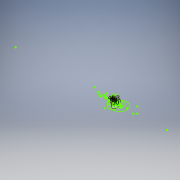
# Autodesk Inventor part: cSkull_meso_WOK_tall_VIS
Saved by Autodesk Inventor 2018 (Build 220112000, 112)
## iProperties
Created: 2018-05-22
Part Number: cSkull_meso_WOK_tall_VIS
Material: Generic
Document SubType Name: Modeling
Designer: McCormick Lab
Density: 1 g/cm^3
Appearance: Default
Author: McCormick Lab
Autodesk Inventor part; units mm, degrees
ref_plane "YZ Plane" through (0, 0, 0) normal (1, 0, 0) x (0, 1, 0)
ref_plane "XZ Plane" through (0, 0, 0) normal (0, 1, 0) x (-1, 0, 0)
ref_plane "XY Plane" through (0, 0, 0) normal (0, 0, 1) x (1, 0, 0)
sketch "Sketch1" plane through (0, 0, 0) normal (1, 0, 0) x (0, 1, 0)
  arc A0 (6, 5) -> (0, 6.4776) centre (1.5083, -0.3184) ccw
  arc A1 (0, 6.4776) -> (-6, 2) centre (-0.0372, 0.2686) ccw
  arc A2 (-6, 2) -> (-5, -3.4628) centre (-1.5043, 0) ccw
  arc A3 (-5, -3.4628) -> (2, -5.5969) centre (1.6627, 5.8444) ccw
  arc A4 (2, -5.5969) -> (6.9353, -3.4628) centre (1.5482, 2.2219) ccw
  arc A5 (6, 5) -> (13, 1) centre (22.0402, 24.9454) ccw
  arc A6 (13, -1) -> (6.9353, -3.4628) centre (16.5953, -18.5517) ccw
  arc A7 (13, -1) -> (13, 1) centre (11.912, 0) ccw
  arc A8 (15.1251, -1.2068) -> (15.1251, 1.1192) centre (13.8597, -0.0438) ccw
  arc A9 (6.9841, 5.7712) -> (15.1251, 1.1192) centre (25.6388, 28.9677) ccw
  arc A10 (6.9841, 5.7712) -> (0.0061, 7.4897) centre (1.7602, -0.414) ccw
  arc A11 (0.0061, 7.4897) -> (-6.9719, 2.2822) centre (-0.0372, 0.2686) ccw
  arc A12 (-6.9719, 2.2822) -> (-5.8089, -4.0711) centre (-1.7435, -0.0438) ccw
  arc A13 (-5.8089, -4.0711) -> (2.3321, -6.5529) centre (1.9397, 6.7532) ccw
  arc A14 (2.3321, -6.5529) -> (8.0718, -4.0711) centre (1.8067, 2.5403) ccw
  arc A15 (15.1251, -1.2068) -> (8.0718, -4.0711) centre (19.3063, -21.6193) ccw
  point P0 (0, 0)
  constraints: 32 point on circle, 16 centre point
sketch "Sketch2" plane through (0, 0, 0) normal (0, 0, 1) x (1, 0, 0)
  arc A0 (4.5893, 15.6275) -> (5.3653, 12.7341) centre (8.4769, 15.1194) ccw
  arc A1 (7.1334, 6.0475) -> (5.3653, 12.7341) centre (-9.3019, 5.2787) ccw
  arc A2 (4, -1) -> (7.1334, 6.0475) centre (-2.3212, 6.0308) ccw
  arc A3 (4, -1) -> (2.2783, -7.605) centre (15.174, -7.4395) ccw
  arc A4 (4.5893, 15.6275) -> (-5.4042, 15.6275) centre (-0.4074, 13.9881) ccw
  arc A5 (-4.7137, -7.4395) -> (2.2783, -7.605) centre (-1.0169, 0.9638) ccw
  arc A6 (-5.4042, 15.6275) -> (-4.7137, -7.4395) centre (15.8945, 4.7212) ccw
  point P0 (0, 0)
  point P1 (16.0644, 6.0537)
  constraints: 14 point on circle, 7 centre point
sketch "Sketch3" plane through (0, 0, 0) normal (0, 0, 1) x (1, 0, 0)
  line L0 (8, 6) -> (8, -9.7213)
  line L1 (8, 6) -> (8, 19.0901)
  arc A0 (8, -9.7213) -> (8, 19.0901) centre (-3.1204, 4.6844) ccw
  point P0 (0, 0)
  constraints: 4 end point, 2 point on circle, 1 centre point, 1 vertical
sketch "Sketch4" plane through (0, 0, 0) normal (0, 0, 1) x (1, 0, 0)
  arc A0 (4, -3) -> (3, -7.466) centre (10.199, -6.733) ccw
  arc A1 (4, -3) -> (7.6292, 3.7812) centre (-12.6955, 10.297) ccw
  arc A2 (7.6292, 3.7812) -> (7, 11) centre (-7.2238, 6.1234) ccw
  arc A3 (7, 11) -> (6.1482, 13) centre (-7.2238, 6.1234) ccw
  arc A4 (5.3976, 15.5783) -> (6.1482, 13) centre (8.6756, 15.1342) ccw
  arc A5 (3, -7.466) -> (9, -9) centre (8, -0.4104) ccw
  arc A6 (11, 18) -> (5.3976, 15.5783) centre (10.5, 11.4654) ccw
  arc A7 (9, -9) -> (11, 18) centre (-69.2967, 10.3738) ccw
  point P0 (0, 0)
  constraints: 16 point on circle, 8 centre point
sketch "Sketch5" plane through (0, 0, 0) normal (1, 0, 0) x (0, 1, 0)
  arc A0 (13, -1.7602) -> (13, 2.0171) centre (12.6189, 0.1284) ccw
  arc A1 (17, 0) -> (13, 2.0171) centre (12.9569, -3.0431) ccw
  arc A2 (13, -1.7602) -> (17, 0) centre (13.7728, 1.9087) ccw
  point P0 (0, 0)
  constraints: 6 point on circle, 3 centre point
sketch "Sketch7" plane through (0, 0, 0) normal (1, 0, 0) x (0, 1, 0)
  circle A0 centre (5, 0.3375) radius 25
  point P0 (0, 0)
  dimension "d10" = 50
  constraints: 1 centre point
  measures "d10" diameter of A0
sketch "Sketch8" plane through (0, 0, 0) normal (0, 0, 1) x (1, 0, 0)
  arc A0 (4.5893, 15.6275) -> (5.3653, 12.7341) centre (8.4769, 15.1194) ccw
  arc A1 (7.1334, 6.0475) -> (5.3653, 12.7341) centre (-9.3019, 5.2787) ccw
  arc A2 (4, -1) -> (7.1334, 6.0475) centre (-2.3212, 6.0308) ccw
  arc A3 (4, -1) -> (2.2783, -7.605) centre (15.174, -7.4395) ccw
  arc A4 (4.5893, 15.6275) -> (-5.4042, 15.6275) centre (-0.4074, 13.9881) ccw
  arc A5 (-4.7137, -7.4395) -> (2.2783, -7.605) centre (-1.0169, 0.9638) ccw
  arc A6 (-5.4042, 15.6275) -> (-4.7137, -7.4395) centre (15.8945, 4.7212) ccw
  point P0 (0, 0)
  constraints: 14 point on circle, 7 centre point
sketch "Sketch9" plane through (0, 0, 0) normal (0, 0, 1) x (1, 0, 0)
  line L0 (2.2936, -15.8564) -> (2.2936, -6.8564)
  arc A0 (2.2936, -6.8564) -> (-3.9962, -9.9765) centre (0.2723, -10.6815) ccw
  arc A1 (-4, -16) -> (2.2936, -15.8564) centre (-0.9465, -11.8394) ccw
  arc A2 (-3.9962, -9.9765) -> (-4, -16) centre (14.3076, -12.9998) ccw
  point P0 (0, 0)
  constraints: 6 point on circle, 3 centre point, 2 end point, 1 tangent
sketch "Sketch10" plane through (0, 0, 0) normal (1, 0, 0) x (0, 1, 0)
  arc A0 (13, -1) -> (13, 1) centre (11.912, 0) ccw
  arc A1 (6, 5) -> (13, 1) centre (22.0402, 24.9454) ccw
  arc A2 (6, 5) -> (0, 6.4776) centre (1.5083, -0.3184) ccw
  arc A3 (0, 6.4776) -> (-6, 2) centre (-0.0372, 0.2686) ccw
  arc A4 (-6, 2) -> (-5, -3.4628) centre (-1.5043, 0) ccw
  arc A5 (-5, -3.4628) -> (2, -5.5969) centre (1.6627, 5.8444) ccw
  arc A6 (2, -5.5969) -> (6.9353, -3.4628) centre (1.5482, 2.2219) ccw
  arc A7 (13, -1) -> (6.9353, -3.4628) centre (16.5953, -18.5517) ccw
  point P0 (0, 0)
  constraints: 16 point on circle, 8 centre point
sketch "Sketch11" plane through (0, 0, 0) normal (0, 0, 1) x (1, 0, 0)
  arc A0 (4, -3) -> (3, -7.466) centre (10.199, -6.733) ccw
  arc A1 (4, -3) -> (7.6292, 3.7812) centre (-12.6955, 10.297) ccw
  arc A2 (7.6292, 3.7812) -> (7, 11) centre (-7.2238, 6.1234) ccw
  arc A3 (7, 11) -> (6.1482, 13) centre (-7.2238, 6.1234) ccw
  arc A4 (5.3976, 15.5783) -> (6.1482, 13) centre (8.6756, 15.1342) ccw
  arc A5 (11, -15) -> (11, 18) centre (-58.5, 1.5) ccw
  arc A6 (3, -7.466) -> (3.1376, -15) centre (85.1776, -9.733) ccw
  arc A7 (6, 24) -> (5.3976, 15.5783) centre (36.0186, 17.6203) ccw
  arc A8 (11, 18) -> (6, 24) centre (2.7033, 16.1694) ccw
  arc A9 (3.1376, -15) -> (11, -15) centre (7.0688, -10.5838) ccw
  arc A10 (5, 24) -> (4.5969, 15.5783) centre (45.756, 17.829) ccw
  arc A11 (-2, 19) -> (4.5969, 15.5783) centre (5.6189, 25.6189) ccw
  arc A12 (5, 24) -> (-2, 19) centre (11.5, 7.5) ccw
  point P0 (0, 0)
  constraints: 26 point on circle, 13 centre point
sketch "Sketch12" plane through (0, 0, 0) normal (1, 0, 0) x (0, 1, 0)
  circle A0 centre (3, 0.2318) radius 20
  circle A1 centre (3, 0.2318) radius 19
  point P0 (0, 0)
  dimension "d21" = 40
  dimension "d22" = 38
  constraints: 2 centre point, 1 coincident
  measures "d21" diameter of A0
  measures "d22" diameter of A1
sketch "Sketch13" plane through (0, 0, 0) normal (0, 0, 1) x (1, 0, 0)
  arc A0 (4.6444, -3) -> (3.6444, -7.466) centre (10.8434, -6.733) ccw
  arc A1 (4.6444, -3) -> (8.2736, 3.7812) centre (-12.0511, 10.297) ccw
  arc A2 (8.2736, 3.7812) -> (7.6444, 11) centre (-6.5793, 6.1234) ccw
  arc A3 (7.6444, 11) -> (6.7926, 13) centre (-6.5793, 6.1234) ccw
  arc A4 (6.042, 15.5783) -> (6.7926, 13) centre (9.3201, 15.1342) ccw
  arc A5 (12.1446, -13.3563) -> (11.6094, 18.8213) centre (-67.1488, 1.418) ccw
  arc A6 (4.5893, 15.6275) -> (5.3653, 12.7341) centre (8.4769, 15.1194) ccw
  arc A7 (7.1334, 6.0475) -> (5.3653, 12.7341) centre (-9.3019, 5.2787) ccw
  arc A8 (4, -1) -> (7.1334, 6.0475) centre (-2.3212, 6.0308) ccw
  arc A9 (4, -1) -> (2.2783, -7.605) centre (15.174, -7.4395) ccw
  arc A10 (-5.4042, 15.6275) -> (-4.7137, -7.4395) centre (15.8945, 4.7212) ccw
  arc A11 (3.6444, -7.466) -> (4.6444, -19) centre (48.1921, -9.4141) ccw
  arc A12 (1, -17) -> (2.2783, -7.605) centre (-20.1318, -9.3402) ccw
  arc A13 (4.5893, 15.6275) -> (4, 28) centre (-90.183, 17.3138) ccw
  arc A14 (6.0097, 28) -> (6.042, 15.5783) centre (472.3708, 23) ccw
  arc A15 (4.6444, -19) -> (12.1446, -13.3563) centre (5.8088, -12.7419) ccw
  arc A16 (11.6094, 18.8213) -> (6.0097, 28) centre (-7.4499, 13.4913) ccw
  arc A17 (-4.7137, -7.4395) -> (1, -17) centre (32.2099, 8.14) ccw
  arc A18 (4, 28) -> (-5.4042, 15.6275) centre (39.2165, -8.5279) ccw
  point P0 (0, 0)
  constraints: 38 point on circle, 19 centre point
sketch "Sketch16" plane through (0, 0, 0) normal (0, 0, 1) x (1, 0, 0)
  arc A0 (7.7852, 10.9763) -> (6.9451, 12.9812) centre (-6.467, 6.1832) ccw
  arc A1 (8.372, 3.7539) -> (7.7852, 10.9763) centre (-6.467, 6.1832) ccw
  arc A2 (4.7031, -3.0059) -> (8.372, 3.7539) centre (-11.9141, 10.3888) ccw
  arc A3 (4.7031, -3.0059) -> (3.6769, -7.4659) centre (10.88, -6.7752) ccw
  arc A4 (6.2096, 15.5639) -> (6.9451, 12.9812) centre (9.485, 15.1006) ccw
  line L0 (3.6769, -7.4659) -> (3.6769, -13)
  line L1 (3.6769, -13) -> (8.7312, -13)
  line L2 (7.1813, -23) -> (8.45, -23) projected
  line L3 (6.2096, 15.5639) -> (6.0634, 19)
  line L4 (6.0634, 19) -> (8.7312, 19)
  line L5 (8.7312, 19) -> (8.7312, -13)
  point P0 (0, 0)
  constraints: 10 end point, 10 point on circle, 5 centre point, 1 parallel, 1 vertical
sketch "Sketch18" plane through (0, 0, 0) normal (0, 1, 0) x (-1, 0, 0)
  arc A0 (0, 16) -> (0, -16) centre (63, 0) ccw
  arc A1 (0, -16) -> (0, 16) centre (-1, 0) ccw
  point P0 (0, 0)
  constraints: 4 point on circle, 2 centre point
sketch "Sketch19" plane through (0, 0, 0) normal (0, 0, 1) x (1, 0, 0)
  arc A0 (0, -13) -> (0, 21.2939) centre (-44.6367, 4.1469) ccw
  arc A1 (0, 21.2939) -> (0, -13) centre (9.2646, 4.1469) ccw
  point P0 (0, 0)
  constraints: 4 point on circle, 2 centre point
sketch "Sketch20" plane through (0, 0, 0) normal (0, 1, 0) x (-1, 0, 0)
  arc A0 (0, 18) -> (0, -21) centre (116.9496, -1.5) ccw
  arc A1 (0, -21) -> (0, 18) centre (-188.5, -1.5) ccw
  point P0 (0, 0)
  constraints: 4 point on circle, 2 centre point
sketch "Sketch21" plane through (0, 0, 0) normal (0, 0, 1) x (1, 0, 0)
  arc A0 (4.5893, 15.6275) -> (5.3653, 12.7341) centre (8.4769, 15.1194) ccw
  arc A1 (7.1334, 6.0475) -> (5.3653, 12.7341) centre (-9.3019, 5.2787) ccw
  arc A2 (4, -1) -> (7.1334, 6.0475) centre (-2.3212, 6.0308) ccw
  arc A3 (4, -1) -> (2.2783, -7.605) centre (15.174, -7.4395) ccw
  arc A4 (-5.4042, 15.6275) -> (-4.7137, -7.4395) centre (15.8945, 4.7212) ccw
  arc A5 (1.6146, -47) -> (2.2783, -7.605) centre (-871.3055, -12.5889) ccw
  arc A6 (-4.7137, -7.4395) -> (1.6146, -47) centre (3.6662, -26.3854) ccw
  arc A7 (6.6047, 48.2766) -> (4.5893, 15.6275) centre (207.8183, 19.4692) ccw
  arc A8 (6.6047, 48.2766) -> (-5.4042, 15.6275) centre (18.1068, 25.5128) ccw
  point P0 (4.9602, 0)
  constraints: 18 point on circle, 9 centre point
sketch "Sketch22" plane through (0, 0, 0) normal (1, 0, 0) x (0, 1, 0)
  arc A0 (12.671, -1.508) -> (10.1452, -2.4415) centre (13.2273, -6.897) ccw
  arc A1 (5.972, -5.9193) -> (10.1452, -2.4415) centre (1.4729, 3.7221) ccw
  arc A2 (-1.0034, -7.134) -> (5.972, -5.9193) centre (0.0411, 7.5036) ccw
  arc A3 (-6.1623, -3.0965) -> (-1.0034, -7.134) centre (-0.5861, -1.2862) ccw
  arc A4 (-5.468, 3.7221) -> (-6.1623, -3.0965) centre (0.6002, -0.3405) ccw
  arc A5 (6.5632, 5.6579) -> (-0.5861, 6.5886) centre (1.6095, -4.4698) ccw
  arc A6 (-0.5861, 6.5886) -> (-5.468, 3.7221) centre (0, 0) ccw
  arc A7 (6.5632, 5.6579) -> (11.3492, 2.8919) centre (22.0985, 27.015) ccw
  arc A8 (14.2401, 1.3463) -> (11.3492, 2.8919) centre (11.1023, -1.0462) ccw
  arc A9 (13.4173, -1.2862) -> (14.2401, 1.3463) centre (12.4465, 0.462) ccw
  arc A10 (12.671, -1.508) -> (13.4173, -1.2862) centre (12.7302, -0.341) ccw
  point P0 (0, 0)
  point P1 (20.1069, -9.3097)
  constraints: 22 point on circle, 11 centre point, 1 tangent
sketch "Sketch23" plane through (0, 0, 0) normal (0, 0, 1) x (1, 0, 0)
  arc A0 (4, -3) -> (3, -7.466) centre (10.199, -6.733) ccw
  arc A1 (4, -3) -> (7.6292, 3.7812) centre (-12.6955, 10.297) ccw
  arc A2 (7.6292, 3.7812) -> (7, 11) centre (-7.2238, 6.1234) ccw
  arc A3 (7, 11) -> (6.1482, 13) centre (-7.2238, 6.1234) ccw
  arc A4 (5.3976, 15.5783) -> (6.1482, 13) centre (8.6756, 15.1342) ccw
  arc A5 (3, -7.466) -> (12.0039, -34.009) centre (74.5087, 1.9925) ccw
  arc A6 (12.0039, -34.009) -> (12.0039, 40.009) centre (-50.8687, 3) ccw
  arc A7 (12.0039, 40.009) -> (5.3976, 15.5783) centre (75.5489, 9.7171) ccw
  point P0 (0, 0)
  constraints: 16 point on circle, 8 centre point
sketch "Sketch24" plane through (0, 0, 0) normal (1, 0, 0) x (0, 1, 0)
  circle A0 centre (4, 0) radius 24.0208
  circle A1 centre (4, 0) radius 54.037
  point P0 (0, 0)
  constraints: 2 centre point, 1 coincident
sketch "Sketch25" plane through (0, 0, 0) normal (0, 0, 1) x (1, 0, 0)
  line L0 (2.9628, -6.7024) -> (3, -28)
  arc A0 (7, 36) -> (4.5756, 19.3965) centre (118.9772, 11.1705) ccw
  arc A1 (5.9839, 23.9235) -> (5.3976, 15.5783) centre (44.4323, 17.0293) ccw
  arc A2 (5.9839, 23.9235) -> (7, 33) centre (-89.9402, 39.2578) ccw
  arc A3 (5.3976, 15.5783) -> (7, 33) centre (-0.8843, 24.9407) ccw
  arc A4 (7, 36) -> (4.5756, 19.3965) centre (13.0884, 26.6322) ccw
  arc A5 (3, -28) -> (2.9628, -6.7024) centre (-3.3961, -17.3623) ccw
  point P0 (0, 0)
  constraints: 12 point on circle, 6 centre point, 2 end point
sketch "Sketch31" plane through (0, 0, 0) normal (1, 0, 0) x (0, 1, 0)
  circle A0 centre (4.1775, 0) radius 24.15
  circle A1 centre (4.1775, 0) radius 23
  point P0 (0, 0)
  dimension "d65" = 46
  dimension "d66" = 48.3
  constraints: 2 centre point, 1 coincident
  measures "d65" diameter of A1
  measures "d66" diameter of A0
sketch "Sketch32" plane through (0, 0, 0) normal (0, 0, 1) x (1, 0, 0)
  arc A0 (4, -1) -> (2.2783, -7.605) centre (15.174, -7.4395) ccw
  arc A1 (4, -1) -> (7.1334, 6.0475) centre (-2.3212, 6.0308) ccw
  arc A2 (7.1334, 6.0475) -> (5.3653, 12.7341) centre (-9.3019, 5.2787) ccw
  arc A3 (4.5893, 15.6275) -> (5.3653, 12.7341) centre (8.4769, 15.1194) ccw
  arc A4 (-5.4042, 15.6275) -> (-4.7137, -7.4395) centre (15.8945, 4.7212) ccw
  arc A5 (1.6146, -47) -> (2.2783, -7.605) centre (-871.3055, -12.5889) ccw
  arc A6 (-4.7137, -7.4395) -> (1.6146, -47) centre (3.6662, -26.3854) ccw
  arc A7 (6.6047, 48.2766) -> (4.5893, 15.6275) centre (207.8183, 19.4692) ccw
  arc A8 (6.6047, 48.2766) -> (-5.4042, 15.6275) centre (18.1068, 25.5128) ccw
  point P0 (0, 0)
  constraints: 18 point on circle, 9 centre point
sketch "Sketch34" plane through (0, 0, 0) normal (0, 0, 1) x (1, 0, 0)
  arc A0 (5, -4) -> (9, 6) centre (-7, 6.6) ccw
  arc A1 (5, -4) -> (4, -8) centre (10.5, -7.5) ccw
  arc A2 (4, -19.9725) -> (4, -8) centre (-95.2669, -13.9862) ccw
  arc A3 (9, 6) -> (6.6308, 15) centre (-16.4523, 4.1118) ccw
  line L0 (6.6308, 15) -> (6.6308, 28.2457)
  arc A4 (4, -19.9725) -> (6.6308, 28.2457) centre (64.4177, 0.9119) ccw
  point P0 (0, 0)
  constraints: 10 point on circle, 5 centre point, 2 end point, 1 vertical
sketch "Sketch35" plane through (0, 0, 0) normal (0, 0, 1) x (1, 0, 0)
  arc A0 (12, -8) -> (-7, -11) centre (15.0455, -88.9545) ccw
  arc A1 (-7, -11) -> (12, -8) centre (3.194, -13.8955) ccw
  point P0 (0, 0)
  constraints: 4 point on circle, 2 centre point
ref_plane "Work Plane16" through (6.6308, 4.1775, 0) normal (1, 0, 0) x (0, 0, -1)
sketch "Sketch36" plane through (6.6308, 4.1775, 0) normal (1, 0, 0) x (0, 0, -1)
  arc A0 (21.5893, 10.8225) -> (-21.5893, 10.8225) centre (0, -0.149) ccw
  arc A1 (20.2947, 10.8225) -> (-20.2947, 10.8225) centre (0, 0) ccw
  line L0 (-21.5893, 10.8225) -> (-20.2947, 10.8225)
  line L1 (-21.5893, 10.8225) -> (-20.2947, 10.8225)
  line L2 (20.2947, 10.8225) -> (21.5893, 10.8225)
  point P0 (0, -4.1775)
  constraints: 6 end point, 4 point on circle, 2 centre point, 1 horizontal
sketch "Sketch37" plane through (0, 0, 0) normal (1, 0, 0) x (0, 1, 0)
  arc A0 (15, 20.2947) -> (6, 22.9277) centre (4.1775, 0) ccw
  arc A1 (15, 21.5893) -> (6, 24.0811) centre (4.9955, 2.9543) ccw
  line L0 (15, 21.5893) -> (15, 20.2947)
  line L1 (15, 21.5893) -> (15, 20.2947)
  line L2 (6, 22.9277) -> (6, 24.0811)
  line L3 (6, 24.0811) -> (6, 22.9277)
  line L4 (15, -20.2947) -> (15, -21.5893) projected
  line L5 (15, -21.5351) -> (15, -20.2947)
  arc A2 (6, -24.0811) -> (15, -21.5893) centre (4.3914, -0.7727) ccw
  arc A3 (6, -22.9277) -> (15, -20.2947) centre (4.1775, 0) ccw
  line L6 (6, -24.0811) -> (6, -22.9277) projected
  line L7 (6, -24.0811) -> (6, -22.9277)
  point P0 (0, 0)
  constraints: 12 end point, 8 point on circle, 4 centre point, 2 collinear, 1 vertical
sketch "Sketch38" plane through (0, 0, 0) normal (0, 0, 1) x (1, 0, 0)
  arc A0 (7.1334, 6) -> (5.3972, 12.671) centre (-9.2641, 5.2939) ccw
  arc A1 (4.5581, 15) -> (5.3972, 12.671) centre (8.676, 15.1681) ccw
  line L0 (0, 15) -> (4.5581, 15) projected
  line L1 (0, 6) -> (7.1334, 6) projected
  arc A2 (4.5581, 15) -> (7.1334, 6) centre (1.4649, 9.2464) ccw
  point P0 (0, 0)
  point P1 (6.4152, 10.1452)
  point P2 (4.945, 13.4173)
  constraints: 8 point on circle, 3 centre point
sketch "Sketch39" plane through (0, 0, 0) normal (0, 0, 1) x (1, 0, 0)
  arc A0 (9, 6) -> (11.63, 15) centre (12.0023, 10.0069) ccw
  arc A1 (9, 6) -> (11.63, 15) centre (-3.4729, 14.5291) ccw
  point P0 (0, 0)
  constraints: 4 point on circle, 2 centre point
sketch "Sketch40" plane through (0, 0, 0) normal (0, 0, 1) x (1, 0, 0)
  arc A0 (1, -11) -> (5, -7) centre (4.0607, -10.0607) ccw
  arc A1 (5, -7) -> (1, -11) centre (6.5, -12.5) ccw
  point P0 (0, 0)
  point P1 (2.963, -6.7889)
  constraints: 4 point on circle, 2 centre point
sketch "Sketch41" plane through (0, 0, 0) normal (0, 0, 1) x (1, 0, 0)
  line L0 (26.7844, 11.2115) -> (14, 17)
  line L1 (14, 17) -> (1.6259, -10.3292)
  line L2 (1.6259, -10.3292) -> (14.4104, -16.1177)
  line L3 (14.4104, -16.1177) -> (26.7844, 11.2115)
  point P0 (0, 0)
  dimension "d87" = 30
  constraints: 8 end point, 2 parallel, 1 perpendicular
  measures "d87" distance between parallel lines of L0 L2
ref_plane "Work Plane13" through (2.4677, -8.47, 20.5733) normal (0.911, -0.4125, 0) x (0, 0, -1)
sketch "Sketch43" plane through (2.4677, -8.47, 20.5733) normal (0.911, -0.4125, 0) x (0, 0, -1)
  line L0 (-2.3543, 15.8761) -> (-3.5078, 15.8761)
  line L1 (-3.5078, 15.8761) -> (-2.3543, 15.8761)
  arc A0 (-3.5078, 15.8761) -> (0.1198, -0.2516) centre (25.1927, 13.8599) ccw
  line L2 (1.4913, -0.2516) -> (0.1198, -0.2516)
  line L3 (0.1198, -0.2516) -> (1.4913, -0.2516)
  line L4 (-1.278, 5.6151) -> (14.6782, 5.6151) projected
  arc A1 (-2.3543, 15.8761) -> (1.4913, -0.2516) centre (22.6187, 13.3086) ccw
  point P0 (20.5733, 6.6981)
  point P1 (1.4551, -0.1819)
  constraints: 8 end point, 5 point on circle, 2 centre point, 1 horizontal
ref_plane "Work Plane14" through (2.964, -7.3739, 19.8888) normal (0.911, -0.4125, 0) x (0, 0, -1)
sketch "Sketch45" plane through (2.964, -7.3739, 19.8888) normal (0.911, -0.4125, 0) x (0, 0, -1)
  line L0 (43.9735, 14.6294) -> (42.8127, 14.6294)
  line L1 (42.8202, 14.6294) -> (43.9735, 14.6294) projected
  arc A0 (40.3423, -1.4549) -> (43.9735, 14.6294) centre (15.2518, 12.6615) ccw
  arc A1 (39, -1.4549) -> (42.8202, 14.6294) centre (15.5968, 12.5994) ccw
  line L2 (40.3423, -1.4549) -> (38.9708, -1.4549)
  line L3 (38.9708, -1.4549) -> (40.3423, -1.4549)
  point P0 (19.8888, 5.4949)
  constraints: 6 end point, 4 point on circle, 2 centre point, 1 collinear, 1 horizontal
sketch "Sketch46" plane through (0, 0, 0) normal (0, 0, 1) x (1, 0, 0)
  arc A0 (8.9982, -11.6413) -> (8.9982, 28.2457) centre (46.0154, 8.3022) ccw
  line L0 (8.9982, 28.2457) -> (8.9982, -11.6413)
  point P0 (0, 0)
  constraints: 2 end point, 2 point on circle, 1 centre point
sketch "Sketch47" plane through (0, 0, 0) normal (0, 0, 1) x (1, 0, 0)
  line L0 (13.5135, 0) -> (-7.3337, 0)
  line L1 (2.3639, -20.2737) -> (9.0424, -23.2975) construction
  line L2 (2.3639, -20.2737) -> (9.0424, -23.2975)
  line L3 (9.0424, -23.2975) -> (9.0424, -24.2545)
  line L4 (9.0424, -24.2545) -> (2.3639, -21.2074)
  line L5 (2.3639, -21.2074) -> (2.3639, -20.2737)
  point P0 (0, 0)
  constraints: 13 end point, 1 horizontal, 1 vertical
sketch "Sketch48" plane through (0, 0, 0) normal (1, 0, 0) x (0, 1, 0)
  line L0 (-7.605, -19.7528) -> (-7.605, 19.6257)
  arc A0 (-7.605, 19.6257) -> (-7.605, -19.7528) centre (1.069, -0.0635) ccw
  point P0 (0, 0)
  constraints: 2 end point, 2 point on circle, 1 centre point
sketch "Sketch49" plane through (0, 0, 0) normal (0, 0, 1) x (1, 0, 0)
  line L0 (2.2936, -7.605) -> (2.2936, -6.8564) projected
  line L1 (2.2936, -6.8564) -> (2.2936, -25.2348)
  arc A0 (2.2936, -6.8564) -> (2.2936, -25.2348) centre (2.131, -16.0456) ccw
  point P0 (0, 0)
  constraints: 2 end point, 2 point on circle, 1 centre point
sketch "Sketch50" plane through (0, 0, 0) normal (0, 0, 1) x (1, 0, 0)
  arc A0 (3.3209, -23.1081) -> (8.9982, 5.953) centre (-195.8612, 30.8887) ccw
  arc A1 (3.3209, -23.1081) -> (3, 48) centre (19.245, 12.5186) ccw
  arc A2 (3, 48) -> (8, 28.2457) centre (151.9378, 75.1876) ccw
  line L0 (8.9982, -11.6413) -> (8.9982, 5.953) projected
  arc A3 (8.9982, 5.953) -> (8, 28.2457) centre (-139.412, 10.4765) ccw
  point P0 (0, 0)
  point P1 (8.9982, 6)
  constraints: 8 point on circle, 4 centre point
sketch "Sketch52" plane through (0, 0, 0) normal (1, 0, 0) x (0, 1, 0)
  line L0 (32, 0) -> (-26, 0)
  arc A0 (32, 0) -> (-26, 0) centre (3, 2.0806) ccw
  point P0 (0, 0)
  constraints: 2 end point, 2 point on circle, 1 centre point, 1 horizontal
sketch "Sketch53" plane through (0, 0, 0) normal (1, 0, 0) x (0, 1, 0)
  arc A0 (13, -1.4779) -> (13, 1.4779) centre (12.9444, 0) ccw
  arc A1 (13, 1.4779) -> (13, -1.4779) centre (15.3831, 0) ccw
  point P0 (0, 0)
  constraints: 4 point on circle, 2 centre point
sketch "Sketch55" plane through (0, 0, 0) normal (0, 0, 1) x (1, 0, 0)
  arc A0 (4.58, 19.7001) -> (6, 11) centre (32.9729, 19.8682) ccw
  arc A1 (4.58, 19.7001) -> (6, 11) centre (11.8372, 16.4186) ccw
  point P0 (0, 0)
  constraints: 4 point on circle, 2 centre point
ref_plane "Work Plane5" through (0, 0, 15) normal (0, 0, 1) x (1, 0, 0)
sketch "Sketch56" plane through (0, 0, 15) normal (0, 0, 1) x (1, 0, 0)
  arc A0 (6.4152, 10.1452) -> (4, 25) centre (-21.1275, 13.2908) ccw
  arc A1 (4, 25) -> (6.4152, 10.1452) centre (20.5376, 20.0651) ccw
  point P0 (0, 0)
  constraints: 4 point on circle, 2 centre point
ref_plane "Work Plane3" through (0, 0, 0) normal (0, 0, 1) x (1, 0, 0)
ref_plane "Work Plane6" through (0, 0, -15) normal (0, 0, 1) x (1, 0, 0)
sketch "Sketch57" plane through (0, 0, -15) normal (0, 0, 1) x (1, 0, 0)
  arc A0 (5.512, 20.9612) -> (4.7992, 23.1043) centre (-21.1275, 13.2908) ccw projected
  arc A1 (6.4152, 10.1452) -> (4.7992, 23.1043) centre (-21.1275, 13.2908) ccw
  arc A2 (4.7992, 23.1043) -> (6.4152, 10.1452) centre (4.6042, 16.4997) ccw
  point P0 (0, 0)
  constraints: 4 point on circle, 2 centre point
ref_plane "Work Plane7" through (0, 0, -15) normal (0, 0, 1) x (1, 0, 0)
sketch "Sketch58" plane through (0, 0, -15) normal (0, 0, 1) x (1, 0, 0)
  arc A0 (4.5821, 19.4868) -> (4.7951, 33.432) centre (-39.5171, 27.1347) ccw
  arc A1 (4.5821, 19.4868) -> (5.6499, 12.1459) centre (32.9729, 19.8682) ccw
  arc A2 (4.7951, 33.432) -> (5.6499, 12.1459) centre (19.8894, 23.3779) ccw
  point P0 (0, 0)
  constraints: 6 point on circle, 3 centre point
ref_plane "Work Plane8" through (0, 0, -15) normal (0, 0, 1) x (1, 0, 0)
sketch "Sketch59" plane through (0, 0, -15) normal (0, 0, 1) x (1, 0, 0)
  arc A0 (4.5821, 19.4868) -> (4.7951, 33.432) centre (-39.5171, 27.1347) ccw
  arc A1 (4.5821, 19.4868) -> (5.6499, 12.1459) centre (32.9729, 19.8682) ccw
  arc A2 (4.7951, 33.432) -> (5.6499, 12.1459) centre (19.8894, 23.3779) ccw
  point P0 (0, 0)
  constraints: 6 point on circle, 3 centre point
sketch "Sketch60" plane through (0, 0, 0) normal (1, 0, 0) x (0, 1, 0)
  line L0 (12.1111, 15) -> (12.1111, 21.5884)
  line L1 (12.1111, 21.5884) -> (12.1111, 15)
  line L2 (20.9612, 15.726) -> (20.9612, 15) projected
  line L3 (20.9612, 15) -> (20.9612, 15.726)
  arc A0 (20.9612, 15.726) -> (12.1111, 21.5884) centre (4.1775, 0) ccw
  line L4 (12.1111, -21.5884) -> (12.1111, -15)
  line L5 (12.1459, -15) -> (12.1111, -21.5884)
  line L6 (20.9612, -15) -> (20.9612, -15.726) projected
  line L7 (20.9612, -15) -> (20.9612, -15.726)
  arc A1 (12.1111, -21.5884) -> (20.9612, -15.726) centre (4.1775, 0) ccw
  line L8 (12.1111, 15) -> (12.1111, 21.5884) projected
  line L9 (22.5441, 15) -> (20.9612, 15) projected
  arc A2 (12.1111, 15) -> (20.9612, 15) centre (16.5362, 45.9173) ccw
  arc A3 (20.9612, -15) -> (12.1111, -15) centre (16.5362, -33.5759) ccw
  point P0 (0, 0)
  constraints: 12 end point, 8 point on circle, 4 centre point, 3 collinear
ref_plane "Work Plane9" through (0, 0, -15) normal (0, 0, 1) x (1, 0, 0)
sketch "Sketch61" plane through (0, 0, -15) normal (0, 0, 1) x (1, 0, 0)
  line L0 (5.6658, 12.1111) -> (6.5691, 12.1111) projected
  line L1 (6.5691, 12.1111) -> (-0.1843, 12.1111)
  line L2 (5.512, 20.9612) -> (-0.1843, 20.9612)
  line L3 (0, 20.9612) -> (4.8126, 20.9612) projected
  arc A0 (-0.1843, 20.9612) -> (-0.1843, 12.1111) centre (11.2781, 16.5362) ccw
  line L4 (6.5691, 12.1111) -> (6.63, 12.1111) projected
  arc A1 (6.5691, 12.1111) -> (5.512, 20.9612) centre (-21.1275, 13.2908) ccw
  point P0 (0, 0)
  constraints: 4 end point, 4 point on circle, 2 centre point
ref_plane "Work Plane10" through (0, 0, -15) normal (0, 0, 1) x (1, 0, 0)
sketch "Sketch62" plane through (0, 0, -15) normal (0, 0, 1) x (1, 0, 0)
  line L0 (6.5691, 12.1111) -> (-0.1843, 12.1111)
  line L1 (5.512, 20.9612) -> (-0.1843, 20.9612)
  arc A0 (-0.1843, 20.9612) -> (-0.1843, 12.1111) centre (11.2781, 16.5362) ccw
  line L2 (4.8126, 20.9612) -> (5.512, 20.9612) projected
  arc A1 (5.512, 20.9612) -> (5.3976, 15.5783) centre (27.7821, 17.7954) ccw
  arc A2 (5.3976, 15.5783) -> (6.1482, 13) centre (8.4638, 15.0726) ccw
  line L3 (6.1482, 13) -> (6.5691, 12.1111)
  point P0 (0, 0)
  point P1 (0, 20.9612)
  constraints: 6 end point, 6 point on circle, 3 centre point
ref_plane "Work Plane12" through (0, 0, 15) normal (0, 0, 1) x (1, 0, 0)
sketch "Sketch65" plane through (0, 0, 15) normal (0, 0, 1) x (1, 0, 0)
  line L0 (0, 12.1111) -> (0, 20.9612)
  line L1 (0, 20.9612) -> (0, 12.1111)
  line L2 (0, 12.1111) -> (5.6659, 12.1111)
  line L3 (0, 12.1111) -> (0, 20.9612) projected
  line L4 (0, 20.9612) -> (4.8105, 20.9612)
  line L5 (0, 20.9612) -> (5.512, 20.9612) projected
  arc A0 (4.8126, 20.9612) -> (4.8105, 16.2544) centre (16.6683, 18.6025) ccw
  arc A1 (4.8105, 16.2544) -> (5.6659, 12.1111) centre (31.8657, 19.6806) ccw
  point P0 (0, 0)
  constraints: 8 end point, 4 point on circle, 2 centre point, 1 point on line
ref_plane "Work Plane11" through (0, 0, 15) normal (0, 0, 1) x (1, 0, 0)
sketch "Sketch67" plane through (0, 0, 15) normal (0, 0, 1) x (1, 0, 0)
  line L0 (0, 12.1111) -> (5.6658, 12.1111)
  line L1 (6.5691, 12.1111) -> (0, 12.1111)
  line L2 (0, 12.1111) -> (0, 20.9612) projected
  line L3 (0, 12.1111) -> (0, 20.9612)
  line L4 (5.512, 20.9612) -> (0, 20.9612)
  arc A0 (5.512, 20.9612) -> (5.3976, 15.5783) centre (27.7821, 17.7954) ccw
  line L5 (6.5691, 12.1111) -> (6.1482, 13)
  arc A1 (5.3976, 15.5783) -> (6.1482, 13) centre (8.4638, 15.0726) ccw
  point P0 (0, 0)
  constraints: 10 end point, 4 point on circle, 2 centre point, 1 collinear, 1 horizontal
ref_plane "Work Plane15" through (6.63, 0, 0) normal (1, 0, 0) x (0, 0, -1)
sketch "Sketch68" plane through (6.63, 0, 0) normal (1, 0, 0) x (0, 0, -1)
  arc A0 (14, 22) -> (14, 11) centre (62.4766, 16.5) ccw
  arc A1 (14, 11) -> (14, 22) centre (11.848, 16.5) ccw
  arc A2 (14, 10) -> (21.6289, 12) centre (11.8491, 33.7543) ccw
  arc A3 (13, 15) -> (14, 10) centre (21, 14) ccw
  arc A4 (21.6289, 12) -> (13, 15) centre (14.4695, 5.3172) ccw
  arc A5 (-21.5884, 12.1111) -> (-13.1641, 12.1459) centre (-17.4061, 19.3527) ccw
  arc A6 (-13.1641, 12.1459) -> (-21.5884, 12.1111) centre (-17.3607, 8.3588) ccw
  arc A7 (-14.3886, 22) -> (-14.4349, 10.6825) centre (-5.1535, 16.3034) ccw
  arc A8 (-14.4349, 10.6825) -> (-14.3886, 22) centre (-35.9078, 16.429) ccw
  point P0 (0, 0)
  constraints: 18 point on circle, 9 centre point
sketch "Sketch69" plane through (0, 0, 0) normal (1, 0, 0) x (0, 1, 0)
  arc A0 (-3, -7.5651) -> (11.0179, -2.9788) centre (0.2424, 6.2404) ccw
  line L0 (-3, -7.5651) -> (-3, -6.6289)
  line L1 (11.0179, -2.9788) -> (11.0179, -1.943)
  arc A1 (11.0179, -1.943) -> (10.1452, -2.6581) centre (12.4245, -4.5498) ccw
  arc A2 (-3, -6.6289) -> (10.1452, -2.6581) centre (0.5731, 5.2863) ccw
  line L2 (-8.9035, 0) -> (17, 0) construction
  arc A3 (11.0179, 2.9788) -> (-3, 7.5651) centre (0.2424, -6.2404) ccw
  line L3 (-3, 7.5651) -> (-3, 6.6289)
  line L4 (11.0179, 2.9788) -> (11.0179, 1.943)
  arc A4 (10.1452, 2.6581) -> (11.0179, 1.943) centre (12.4245, 4.5498) ccw
  arc A5 (10.1452, 2.6581) -> (-3, 6.6289) centre (0.5731, -5.2863) ccw
  point P0 (0, 0)
  point P1 (6.0475, -5.8837)
  constraints: 13 point on circle, 10 end point, 8 symmetric about line, 6 centre point, 1 tangent, 1 vertical, 3 other
sketch "Sketch70" plane through (0, 0, 0) normal (0, 0, 1) x (1, 0, 0)
  arc A0 (4, -3) -> (7.812, 5.972) centre (-6.9875, 6.9641) ccw
  arc A1 (4, -3) -> (8, -3) centre (6, 0.2231) ccw
  arc A2 (8, -3) -> (7.812, 5.972) centre (-95.4852, -0.6804) ccw
  arc A3 (7.8, 6.0475) -> (6.9938, 11.0179) centre (-4.9894, 6.5238) ccw
  arc A4 (7.8, 6.0475) -> (6.9938, 11.0179) centre (7.8859, 8.612) ccw
  arc A5 (3.0655, -3) -> (5.6658, 12.1111) centre (-16.4907, 8.1445) ccw
  line L0 (3.0655, -3) -> (4, -3) projected
  arc A6 (5.6658, 12.1111) -> (3.0655, -3) centre (0.9123, 5.1498) ccw
  constraints: 14 point on circle, 7 centre point
sketch "Sketch71" plane through (0, 0, 0) normal (0, 0, 1) x (1, 0, 0)
  line L0 (21.3234, 1.813) -> (-3.8328, 3.9894)
  line L1 (6.7281, 29.5792) -> (31.9548, 41.3881)
  line L2 (2.1762, -23.0341) -> (25, -39)
  line L3 (2.1762, -23.0341) -> (2.3639, -21.5054)
  line L4 (2.3639, -21.5054) -> (3.7434, -22.1348)
  line L5 (3.7434, -22.1348) -> (4.2532, -20)
  line L6 (4.2532, -20) -> (3.0537, -20.1909)
  line L7 (3.0537, -20.1909) -> (3, -18)
  line L8 (3, -18) -> (6, -19)
  line L9 (6, -19) -> (5.7028, -22.6912)
  line L10 (5.7028, -22.6912) -> (25, -36)
  line L11 (25, -39) -> (25, -36)
  line L12 (6.7281, 29.5792) -> (6.7281, 28.625)
  line L13 (6.7281, 28.625) -> (8.2975, 28.625)
  line L14 (8.2975, 28.625) -> (8.7453, 26.5871)
  line L15 (8.7453, 26.5871) -> (6.7281, 26.5871)
  line L16 (6.7281, 26.5871) -> (6.7281, 25.1274)
  line L17 (6.7281, 25.1274) -> (9.7835, 25.1274)
  line L18 (9.7835, 25.1274) -> (9.4996, 29.1021)
  line L19 (9.4996, 29.1021) -> (31.9548, 38.8479)
  line L20 (31.9548, 41.3881) -> (31.9548, 38.8479)
  point P0 (0, 0)
  constraints: 42 end point, 4 vertical, 3 horizontal, 2 symmetric about line
revolve "Revolution4" add sketch "Sketch71" angle 180 mid plane about axis through (21.3234, 1.813, 0) along (-0.9963, 0.0862, 0)
body "Solid1"
